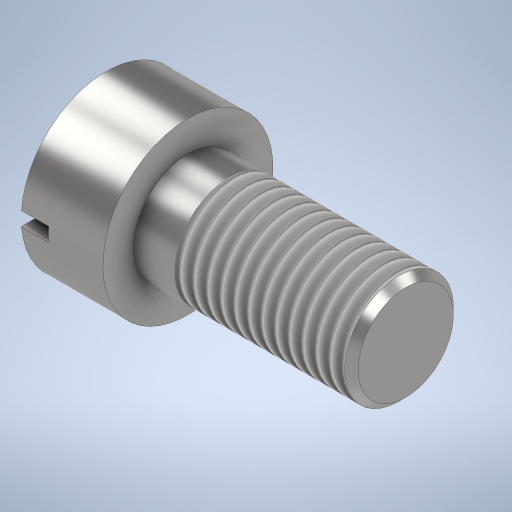
# Autodesk Inventor part: M16bolt
Saved by Autodesk Inventor 2024 (Build 280153000, 153)
## iProperties
Created: 2023-11-09
Part Number: M16bolt
Material: Iron, Malleable
Document SubType Name: Modeling
Designer: Admin
Density: 7.15 g/cm^3
Appearance: Semi-Polished
Author: Admin
Autodesk Inventor part; units mm, degrees
ref_plane "YZ Plane" through (0, 0, 0) normal (1, 0, 0) x (0, 1, 0)
ref_plane "XZ Plane" through (0, 0, 0) normal (0, 1, 0) x (-1, 0, 0)
ref_plane "XY Plane" through (0, 0, 0) normal (0, 0, 1) x (1, 0, 0)
sketch "Sketch1" plane through (0, 0, 0) normal (1, 0, 0) x (0, 1, 0)
  circle A0 centre (0, 0) radius 12.5
  circle A1 centre (0, 0) radius 8
  dimension "d0" = 25
  dimension "d1" = 16
  constraints: 2 centre point, 2 coincident
  measures "d0" diameter of A0
  measures "d1" diameter of A1
extrude "Extrusion1" add sketch "Sketch1" against normal blind 12 contours A0 | A1
extrude "Extrusion2" add sketch "Sketch1" along normal blind 32 contours A1
chamfer "Chamfer1" distance 1 angle 45 1 edges at (32, -8, 0) measured on face at (32, 0.9456, 2.4934)
thread "Thread1" size "M16x2" class "6g" standard "ANSI Metric M Profile" length 25
sketch "Sketch2" plane through (-12, 0, 0) normal (-1, 0, 0) x (0, 0, 1)
  circle A0 centre (0, 0) radius 12.5 construction
  line L0 (-17.5, 0) -> (17.5, 0) construction
  line L1 (12.4599, -1) -> (12.4599, 1) construction
  line L2 (-12.4599, 1) -> (-12.4599, -1) construction
  line L3 (-12.8, 1) -> (-12.8, -1)
  line L4 (12.7599, -1) -> (12.7599, 1)
  line L5 (-12.8, -1) -> (12.7599, -1)
  line L6 (12.7599, -1) -> (12.7599, 1)
  line L7 (12.7599, 1) -> (-12.8, 1)
  line L8 (-12.8, 1) -> (-12.8, -1)
  point P0 (0, 1)
  point P1 (0, -1)
  point P2 (12.5, 0)
  point P3 (12.5, 0)
  point P4 (-12.5, 0)
  point P5 (-12.5, 0)
  dimension "d11" = 2
  dimension "d14" = 0.3
  dimension "d15" = 0.3
  dimension "d16" = 1
  dimension "d17" = 1
  dimension "d18" = 25.5599
  dimension "d19" = 1
  dimension "d20" = 0
  dimension "d21" = 0
  dimension "d22" = 1
  dimension "d23" = 1
  dimension "d24" = 0
  dimension "d25" = 1
  constraints: 16 end point, 6 parallel, 4 horizontal alignment, 1 coincident, 1 horizontal, 1 perpendicular, 1 symmetric about line, 1 vertical alignment, 9 other
  measures "d11" distance of point (0, -1) point (0, 1)
  measures "d14" distance between parallel lines of L1 L4
  measures "d15" distance from line of point (-12.5, 0) L3
  measures "d16" distance between parallel lines of L7 L0
  measures "d17" distance between parallel lines of L5 L0
  measures "d18" distance between parallel lines of L4 L3
  measures "d19" distance from line of L4.start L0
  measures "d20" distance from line of point (12.5, 0) L0
  measures "d21" distance from line of point (12.5, 0) L0
  measures "d22" distance from line of L1.start L0
  measures "d23" distance from line of L2.start L0
  measures "d24" distance from line of point (-12.5, 0) L0
  measures "d25" distance from line of L3.start L0
extrude "Extrusion5" cut sketch "Sketch2" against normal blind 4
body "Solid1"
